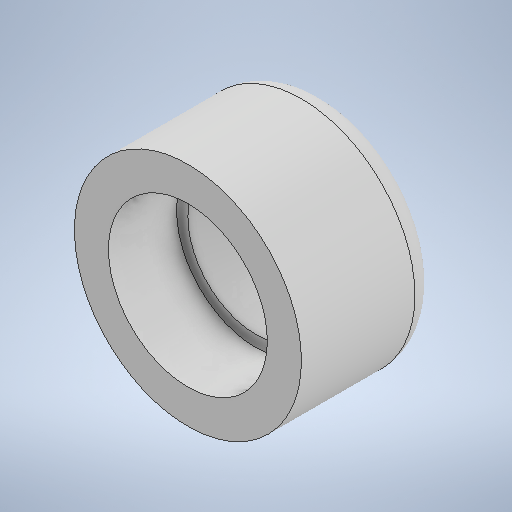
# Autodesk Inventor part: 26b
Saved by Autodesk Inventor 2025.1 (Build 291241000, 241)
## iProperties
Created: 2024-09-13
Part Number: 26b
Material: Generisch
Document SubType Name: Modeling
Designer: ffogue
Density: 1 g/cm^3
Appearance: Vorgabe
Author: ffogue
Autodesk Inventor part; units mm, degrees
ref_plane "YZ Plane" through (0, 0, 0) normal (1, 0, 0) x (0, 1, 0)
ref_plane "XZ Plane" through (0, 0, 0) normal (0, 1, 0) x (-1, 0, 0)
ref_plane "XY Plane" through (0, 0, 0) normal (0, 0, 1) x (1, 0, 0)
sketch "Sketch1" plane through (0, 0, 0) normal (0, 0, 1) x (1, 0, 0)
  line L0 (0, 0) -> (0, 6)
  line L1 (0, 6) -> (5, 6)
  line L2 (5, 6) -> (5, 0)
  line L3 (5, 0) -> (3.5, 0)
  line L4 (3.5, 0) -> (3.5, 3)
  line L5 (3.5, 3) -> (0, 3)
  point P0 (4.25, 0)
  dimension "d0" = 7
  dimension "d1" = 10
  dimension "d2" = 3
  dimension "d3" = 6
  constraints: 12 end point, 4 perpendicular, 2 midpoint, 1 horizontal alignment, 1 vertical
  measures "d0" diameter of L4 L0
  measures "d1" diameter of L2 L0
  measures "d2" distance from line of point (4.25, 0) L5
  measures "d3" distance between parallel lines of L3 L1
revolve "Revolution1" add sketch "Sketch1" angle 360 about axis through (0, 0, 0) along (0, 1, 0)
sketch "Sketch2" plane through (0, 3, 0) normal (0, -1, 0) x (1, 0, 0)
  circle A0 centre (0, 0) radius 3.5 projected
  constraints: 1 coincident
hole "Hole1" at (0, 3, 0) direction (0, 1, 0) diameter 3 depth 3 countersink diameter 6 countersink angle 90
fillet "Fillet1" radius 1 1 edges at (-5, 6, 0)
body "Solid1"
